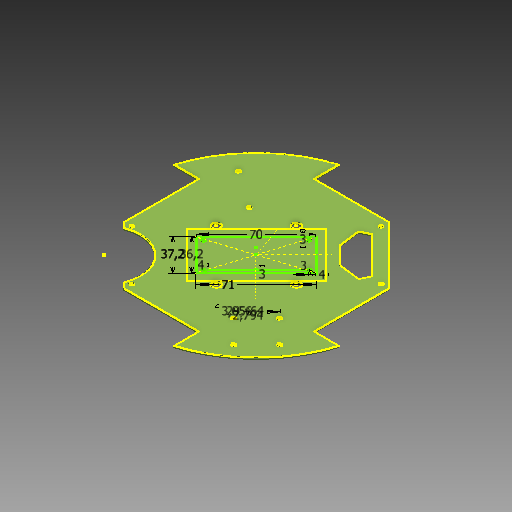
# Autodesk Inventor part: Board1.2
Saved by Autodesk Inventor 2020 (Build 240168000, 168)
## iProperties
Created: 2024-09-20
Part Number: Board1.2
Material: Типовые
Document SubType Name: Modeling
Designer: Ivan
Density: 1 g/cm^3
Appearance: Оливково-зеленый
Author: Ivan
Autodesk Inventor part; units mm, degrees
ref_plane "YZ Plane" through (0, 0, 0) normal (1, 0, 0) x (0, 1, 0)
ref_plane "XZ Plane" through (0, 0, 0) normal (0, 1, 0) x (-1, 0, 0)
ref_plane "XY Plane" through (0, 0, 0) normal (0, 0, 1) x (1, 0, 0)
sketch "Эскиз1" plane through (0, 0, 0) normal (0, 1, 0) x (-1, 0, 0)
  line L0 (-42.002343, -27.440424) -> (-27.440424, -42.002343)
  line L1 (-27.440424, -42.002343) -> (-25.169576, -59.537657)
  line L2 (-25.169576, -59.537657) -> (-32.692388, -63.237612)
  line L3 (-32.692388, -63.237612) -> (-63.237612, -32.692388)
  line L4 (-63.237612, -32.692388) -> (-59.537657, -25.169576)
  line L5 (-59.537657, -25.169576) -> (-42.002343, -27.440424)
  circle A0 centre (-72.43, 16) radius 3.3 construction
  circle A1 centre (44.87, -82.901522) radius 3.3 construction
  circle A2 centre (42.22, 16) radius 3.3
  circle A3 centre (-44.87, 82.901522) radius 3.3 construction
  circle A4 centre (-42.22, 16) radius 3.3 construction
  circle A5 centre (-82.901522, 44.87) radius 3.3 construction
  circle A6 centre (-16, 42.22) radius 3.3 construction
  circle A7 centre (72.43, -16) radius 3.3 construction
  circle A8 centre (16, -72.43) radius 3.3 construction
  circle A9 centre (-16, -72.43) radius 3.3 construction
  circle A10 centre (-42.22, -16) radius 3.3 construction
  circle A11 centre (16, -42.22) radius 3.3 construction
  circle A12 centre (16, 42.22) radius 3.3
  circle A13 centre (16, 72.43) radius 3.3 construction
  circle A14 centre (42.22, -16) radius 3.3 construction
  circle A15 centre (72.43, 16) radius 3.3 construction
  circle A16 centre (-16, 72.43) radius 3.3 construction
  circle A17 centre (82.901522, -44.87) radius 3.3 construction
  circle A18 centre (-16, -42.22) radius 3.3 construction
  circle A19 centre (-72.43, -16) radius 3.3 construction
  line L6 (31, 78.772353) -> (-31, 78.772353)
  line L7 (-31, 78.772353) -> (-31, 99.272353)
  arc A20 (-31, 99.272353) -> (-99.272353, 31) centre (0, 0) ccw
  line L8 (-99.272353, 31) -> (-78.772353, 31)
  line L9 (-78.772353, 31) -> (-78.772353, -31)
  line L10 (-78.772353, -31) -> (-99.272353, -31)
  arc A21 (-99.272353, -31) -> (-98.086264, -34.57) centre (0, 0) ccw
  arc A22 (-34.57, -98.086264) -> (-98.086264, -34.57) centre (-109.02125, -109.02125) ccw
  arc A23 (-34.57, -98.086264) -> (-31, -99.272353) centre (0, 0) ccw
  line L11 (-31, -99.272353) -> (-31, -78.772353)
  line L12 (-31, -78.772353) -> (31, -78.772353)
  line L13 (31, -78.772353) -> (31, -99.272353)
  arc A24 (31, -99.272353) -> (99.272353, -31) centre (0, 0) ccw
  line L14 (99.272353, -31) -> (78.772353, -31)
  line L15 (78.772353, -31) -> (78.772353, 31)
  line L16 (78.772353, 31) -> (99.272353, 31)
  arc A25 (99.272353, 31) -> (98.086264, 34.57) centre (0, 0) ccw
  arc A26 (34.57, 98.086264) -> (98.086264, 34.57) centre (109.02125, 109.02125) ccw
  arc A27 (34.57, 98.086264) -> (31, 99.272353) centre (0, 0) ccw
  line L17 (31, 99.272353) -> (31, 78.772353)
  circle A28 centre (31, 72.43) radius 1.5
  circle A29 centre (72.43, 31) radius 1.5
  circle A30 centre (0, 0) radius 20
  circle A31 centre (-72.43, -31) radius 1.5
  circle A32 centre (-31, -72.43) radius 1.5
  line L18 (-55.861436, 32.526912) -> (-79.195959, 55.861436)
  line L19 (-79.195959, 55.861436) -> (-55.861436, 79.195959)
  line L20 (-55.861436, 79.195959) -> (-32.526912, 55.861436)
  line L21 (-32.526912, 55.861436) -> (-55.861436, 32.526912)
  line L22 (48.313848, -22.45283) -> (80.459207, -54.598189)
  line L23 (80.459207, -54.598189) -> (54.598189, -80.459207)
  line L24 (54.598189, -80.459207) -> (22.45283, -48.313848)
  line L25 (22.45283, -48.313848) -> (48.313848, -22.45283)
  line L26 (31, 78.772353) -> (78.772353, 31)
  circle A33 centre (31, 72.43) radius 3.5 construction
  circle A34 centre (72.43, 31) radius 1.5 construction
  circle A35 centre (72.43, 31) radius 3.5 construction
  arc A36 (35.373192, 74.399161) -> (74.399161, 35.373192) centre (63.193264, 63.193264) ccw
  line L27 (-47.729708, -10.253048) -> (10.253048, 47.729708)
  line L28 (10.253048, 47.729708) -> (47.729708, 10.253048)
  line L29 (47.729708, 10.253048) -> (-10.253048, -47.729708)
  line L30 (-10.253048, -47.729708) -> (-47.729708, -10.253048)
  line L31 (-32.526912, 55.861436) -> (-55.861436, 32.526912) construction
  line L32 (-47.729708, -10.253048) -> (47.729708, 10.253048) construction
  line L33 (-78.772353, -31) -> (-31, -78.772353)
  dimension "d0" = 7
  dimension "d1" = 7
  dimension "d2" = 82
  dimension "d3" = 53
  constraints: 68 end point, 37 centre point, 18 point on circle, 4 coincident, 3 parallel, 2 point on line, 2 tangent, 1 midpoint, 1 perpendicular
  measures "d0" diameter of A33
  measures "d1" diameter of A35
  measures "d2" distance of L28.end L29.end
  measures "d3" distance of L27.end L28.end
extrude "Выдавливание1" add sketch "Эскиз1" along normal blind 1.6 contours A2 L28 | L28 A12 | L26 A36 L15 L14 A24 L13 L12 L33 L9 L8 A20 L7 L6 | L18 L19 L20 L21 | L22 L23 L24 L25 picked at (43.146155, 15.474263) picked at (17.150343, 42.083412)
sketch "Эскиз2" plane through (0, 0, 0) normal (0, 1, 0) x (1, 0, 0)
  circle A0 centre (26.769578, -48.318655) radius 1.397
  circle A1 centre (47.603772, -27.484461) radius 1.397
  line L0 (47.603772, -27.484461) -> (26.769578, -48.318655) construction
  line L1 (22.45283, -48.313848) -> (24.613608, -50.474625) construction
  line L2 (26.769578, -48.318655) -> (24.613608, -50.474625) construction
  line L3 (-47.729708, -10.253048) -> (10.253048, 47.729708)
  line L4 (47.729708, 10.253048) -> (-10.253048, -47.729708)
  point P0 (-22.45283, 48.313848)
  point P1 (-79.195959, 55.861436)
  point P2 (79.195959, -55.861436)
  dimension "d6" = 3.0558
  dimension "d8" = 29.464
  dimension "d9" = 2.794
  constraints: 6 end point, 2 centre point, 1 collinear, 1 equal radius, 1 perpendicular
  measures "d6" distance from line of L0 L1.start
  measures "d8" distance of L0.start L0.end
  measures "d9" diameter of A0
sketch "Эскиз4" plane through (0, 1.6, 0) normal (0, 1, 0) x (1, 0, 0)
  arc A0 (75.513396, -56.886374) -> (75.513396, -52.643733) centre (73.392076, -54.765053) ccw
  line L0 (75.513396, -52.643733) -> (57.12862, -34.258957)
  arc A1 (57.12862, -34.258957) -> (52.885979, -34.258957) centre (55.007299, -36.380277) ccw
  line L1 (52.885979, -34.258957) -> (34.501203, -52.643733)
  arc A2 (34.501203, -52.643733) -> (34.501203, -56.886374) centre (36.622523, -54.765053) ccw
  line L2 (34.501203, -56.886374) -> (52.885979, -75.27115)
  arc A3 (52.885979, -75.27115) -> (57.12862, -75.27115) centre (55.007299, -73.14983) ccw
  line L3 (57.12862, -75.27115) -> (75.513396, -56.886374)
  circle A4 centre (62.785474, -48.754646) radius 0.5
  circle A5 centre (55.007299, -73.856937) radius 1.6
  circle A6 centre (74.099182, -54.765053) radius 1.6
  circle A7 centre (55.007299, -35.67317) radius 1.6
  circle A8 centre (61.017707, -39.915811) radius 0.5
  circle A9 centre (55.714406, -41.683578) radius 0.5
  circle A10 centre (57.482173, -43.451345) radius 0.5
  circle A11 centre (59.24994, -45.219112) radius 0.5
  circle A12 centre (61.017707, -46.986879) radius 0.5
  circle A13 centre (43.693591, -64.310995) radius 0.5
  circle A14 centre (41.925824, -62.543228) radius 0.5
  circle A15 centre (62.785474, -41.683578) radius 0.5
  circle A16 centre (59.24994, -38.148044) radius 0.5
  circle A17 centre (53.946639, -39.915811) radius 0.5
  circle A18 centre (35.915416, -54.765053) radius 1.6
  circle A19 centre (40.158057, -60.775461) radius 0.5
  circle A20 centre (38.39029, -59.007694) radius 0.5
  circle A21 centre (64.553241, -50.522413) radius 0.5
  circle A22 centre (66.321008, -45.219112) radius 0.5
  circle A23 centre (64.553241, -43.451345) radius 0.5
  circle A24 centre (68.088775, -46.986879) radius 0.5
  circle A25 centre (69.856542, -48.754646) radius 0.5
  circle A26 centre (71.624309, -50.522413) radius 0.5
  line L4 (47.729708, 10.253048) -> (-10.253048, -47.729708)
  line L5 (18.73833, -18.73833) -> (73.539105, -73.539105) construction
  arc A27 (31, -99.272353) -> (99.272353, -31) centre (0, 0) ccw
  line L6 (-31, -78.772353) -> (31, -78.772353)
  line L7 (78.772353, -31) -> (31, -78.772353) construction
  point P0 (55.007299, -54.765053)
  point P1 (54.886176, -54.886176)
  constraints: 27 centre point, 12 end point, 9 point on circle, 2 midpoint, 1 point on line
extrude "Выдавливание4" cut sketch "Эскиз4" against normal through all contours A5 | A6 | A7 | A18
sketch "Эскиз5" plane through (0, 0, 0) normal (0, -1, 0) x (1, 0, 0)
  circle A0 centre (-37.246198, -31.292358) radius 1.6
  circle A1 centre (-67.882251, -53.033009) radius 1.6
  arc A2 (99.272353, 31) -> (31, 99.272353) centre (0, 0) ccw
  constraints: 3 centre point, 2 point on circle
extrude "Выдавливание5" cut sketch "Эскиз5" against normal through all
sketch "Эскиз6" plane through (0, 1.6, 0) normal (0, 1, 0) x (1, 0, 0)
  circle A0 centre (49.151483, 117.512898) radius 1.65
  circle A1 centre (49.151483, 117.512898) radius 3.35
  circle A2 centre (3.90139, 156.848367) radius 1.65
  circle A3 centre (79.999989, 152.999936) radius 1.65
  circle A4 centre (34.74993, 192.33537) radius 1.65
  circle A5 centre (41.950689, 154.924131) radius 41.494038
  line L0 (45.976694, 118.582111) -> (51.702547, 119.684205)
  arc A6 (39.303109, 113.514645) -> (45.976694, 118.582111) centre (26.737362, 136.991182) ccw
  arc A7 (51.702547, 119.684205) -> (59.780333, 117.456035) centre (62.733836, 143.919668) ccw
  arc A8 (78.499345, 155.995027) -> (82.588741, 163.308869) centre (57.591924, 172.485191) ccw
  circle A9 centre (79.999989, 152.999936) radius 3.35
  arc A10 (81.535526, 142.482434) -> (78.204844, 150.171517) centre (55.740492, 135.874711) ccw
  arc A11 (5.402031, 153.853275) -> (1.312636, 146.539393) centre (26.309482, 137.363149) ccw
  circle A12 centre (3.90139, 156.848367) radius 3.35
  arc A13 (2.365865, 167.365871) -> (5.696538, 159.676785) centre (28.160906, 173.973566) ccw
  arc A14 (32.198864, 190.164066) -> (24.121078, 192.392253) centre (21.16753, 165.928649) ccw
  circle A15 centre (34.74993, 192.33537) radius 3.35
  arc A16 (44.598268, 196.333616) -> (37.924718, 191.266155) centre (57.164078, 172.857113) ccw
  line L1 (39.303109, 113.514645) -> (59.780333, 117.456035) construction
  line L2 (-47.022601, -10.253048) -> (10.253048, 47.022601) construction
  line L3 (2.365865, 167.365871) -> (59.780333, 117.456035) construction
  line L4 (24.121036, 192.392233) -> (81.535512, 142.48239) construction
  line L5 (1.312636, 146.539393) -> (44.598268, 196.333616) construction
  line L6 (82.588741, 163.308869) -> (39.303109, 113.514645) construction
  circle A17 centre (41.950689, 154.924131) radius 38.097924 construction
  line L7 (45.976694, 118.582111) -> (46.911064, 113.727652) construction
  line L8 (78.204844, 150.171517) -> (78.499345, 155.995027) construction
  line L9 (41.950689, 154.924131) -> (79.999989, 152.999936) construction
  line L10 (41.950689, 154.924131) -> (34.74993, 192.33537) construction
  line L11 (41.950689, 154.924131) -> (3.90139, 156.848367) construction
  line L12 (5.696538, 159.676785) -> (5.402031, 153.853275) construction
  line L13 (32.198864, 190.164066) -> (37.924718, 191.266155) construction
  line L14 (41.950689, 154.924131) -> (49.151483, 117.512898) construction
  circle A18 centre (-37.822435, 4.573567) radius 3.3
  circle A19 centre (-4.573567, 37.822435) radius 3.3
  circle A20 centre (4.573567, -37.822435) radius 3.3
  circle A21 centre (37.822435, -4.573567) radius 3.3
  circle A22 centre (16, -49.72) radius 3.3
  line L15 (-37.822435, 4.573567) -> (-4.573567, 37.822435) construction
  line L16 (4.573567, -37.822435) -> (37.822435, -4.573567) construction
  line L17 (-21.198001, 21.198001) -> (21.198001, -21.198001) construction
  line L18 (-4.573567, 37.822435) -> (37.822435, -4.573567) construction
  point P0 (-47.616756, 71.930474)
  point P1 (-60.382397, 55.652797)
  point P2 (-60.382397, 22.39343)
  point P3 (-47.616756, 6.115753)
  point P4 (2.783098, 6.115753)
  point P5 (15.548739, 22.39343)
  point P6 (15.244077, 55.858669)
  point P7 (2.910415, 71.585522)
  point P8 (0, 0)
  point P9 (-47.616756, 71.930474)
  point P10 (-60.382397, 55.652797)
  point P11 (-60.382397, 22.39343)
  point P12 (-47.616756, 6.115753)
  point P13 (2.783098, 6.115753)
  point P14 (15.548739, 22.39343)
  point P15 (15.244077, 55.858669)
  point P16 (2.910415, 71.585522)
  point P17 (0, 0)
  dimension "d45" = 82.98808
  dimension "d43" = 3.3
  dimension "d44" = 6.7
  dimension "d46" = 26.62791
  dimension "d47" = 20.47722
  dimension "d48" = 3.71477
  dimension "d49" = 33.16031
  dimension "d50" = 50.33796
  dimension "d51" = 16.58016
  dimension "d52" = 25.16898
  dimension "d53" = 10.42652
  dimension "d54" = 10.42652
  dimension "d55" = 10.42652
  dimension "d56" = 10.42652
  dimension "d57" = 10.42652
  dimension "d58" = 10.42652
  dimension "d59" = 59.957
  dimension "d60" = 47.021
  constraints: 38 end point, 28 point on circle, 22 centre point, 13 equal radius, 9 perpendicular, 6 coincident, 4 equal length, 4 parallel, 3 midpoint, 1 tangent, 12 other
  measures "d43" diameter of A0
  measures "d44" diameter of A1
  measures "d46" radius of A6
  measures "d47" horizontal distance of L1.end L1.start
  measures "d48" distance from line of L1 L0.start
  measures "d49" distance from line of L4 L3.start
  measures "d50" distance from line of L5 L6.start
  measures "d51" distance from line of L3 point (41.951, 154.924)
  measures "d52" distance from line of L5 point (41.951, 154.924)
  measures "d53" distance from line of L9 L6.start
  measures "d54" distance from line of L9 A10.start
  measures "d55" distance from line of L10 A14.end
  measures "d56" distance from line of L10 L5.end
  measures "d57" distance from line of L11 L3.start
  measures "d58" distance from line of L14 L1.end
  measures "d59" distance from line of L15 L16.end
  measures "d60" distance from line of L18 L15.start
extrude "Выдавливание6" cut sketch "Эскиз6" against normal blind 10 contours A18 | A19 | A20 | A21
sketch "Эскиз7" plane through (0, 1.6, 0) normal (0, 1, 0) x (1, 0, 0)
  line L0 (-38.254477, -11.950105) -> (-11.950105, -38.254477)
  line L1 (-11.950105, -38.254477) -> (38.254477, 11.950105)
  line L2 (38.254477, 11.950105) -> (11.950105, 38.254477)
  line L3 (11.950105, 38.254477) -> (-38.254477, -11.950105)
  line L4 (-38.254477, -11.950105) -> (38.254477, 11.950105) construction
  line L5 (-11.950105, -38.254477) -> (11.950105, 38.254477) construction
  line L6 (47.022601, 10.253048) -> (-10.253048, -47.022601) construction
  line L7 (-47.729708, -10.253048) -> (10.253048, 47.729708)
  line L8 (-10.253048, -47.729708) -> (-47.729708, -10.253048)
  line L9 (10.253048, 47.729708) -> (47.729708, 10.253048)
  line L10 (47.729708, 10.253048) -> (-10.253048, -47.729708)
  line L11 (-38.254477, -11.950105) -> (-11.950105, -38.254477)
  line L12 (-11.950105, -38.254477) -> (38.254477, 11.950105)
  line L13 (38.254477, 11.950105) -> (11.950105, 38.254477)
  line L14 (11.950105, 38.254477) -> (-38.254477, -11.950105)
  line L15 (-38.254477, -11.950105) -> (38.254477, 11.950105) construction
  line L16 (-11.950105, -38.254477) -> (11.950105, 38.254477) construction
  line L17 (47.022601, 10.253048) -> (-10.253048, -47.022601) construction
  line L18 (37.54737, 11.950105) -> (11.950105, 37.54737)
  line L19 (11.950105, 37.54737) -> (-37.54737, -11.950105)
  line L20 (-37.54737, -11.950105) -> (-11.950105, -37.54737)
  line L21 (-11.950105, -37.54737) -> (37.54737, 11.950105)
  line L22 (37.54737, 11.950105) -> (-37.54737, -11.950105) construction
  line L23 (32.597623, 11.242998) -> (-11.242998, -32.597623)
  line L24 (0, 0) -> (31.732181, -31.732181) construction
  circle A0 centre (32.597623, 11.242998) radius 1.5
  line L25 (0, 0) -> (31.732181, 31.732181) construction
  line L26 (0, 0) -> (-9.9, 29) construction
  circle A1 centre (11.242998, 32.597623) radius 1.5
  circle A2 centre (-11.242998, -32.597623) radius 1.5
  circle A3 centre (-32.597623, -11.242998) radius 1.5
  point P0 (0, 0)
  point P1 (0, 0)
  point P2 (10.677312, -10.677312)
  point P3 (-4.979708, 4.979708)
  point P4 (0, 0)
  dimension "d63" = 37.2
  dimension "d64" = 71
  dimension "d67" = 37.2
  dimension "d68" = 71
  dimension "d69" = 36.2
  dimension "d70" = 70
  dimension "d71" = 4
  dimension "d72" = 3
  dimension "d73" = 3
  dimension "d74" = 3
  dimension "d75" = 4
  constraints: 46 end point, 10 parallel, 9 midpoint, 5 coincident, 4 centre point, 4 perpendicular, 3 symmetric about line, 2 point on line, 4 other
  measures "d63" distance of L0.start L0.end
  measures "d64" distance from line of L0 L1.end
  measures "d67" distance of L11.start L11.end
  measures "d68" distance from line of L11 L12.end
  measures "d69" distance of L20.end L19.end
  measures "d70" distance of L19.end L18.end
  measures "d71" distance from line of L18 L23.start
  measures "d72" distance from line of L21 point (10.677, -10.677)
  measures "d73" diameter of A0
  measures "d74" distance from line of L19 A1.centre
  measures "d75" distance from line of L20 L23.end
extrude "Выдавливание8" add sketch "Эскиз7" against normal up to surface (1.6 mm away) contours L3 L2 L1 L0 | L7 L9 L10 L8 | L21 L20 L19 L18 | A0 | A1 | A2 | A3
hole "Отверстие1" at (-32.597623, 1.6, 11.242998) at (11.242998, 1.6, -32.597623) at (32.597623, 1.6, -11.242998) at (-11.242998, 1.6, 32.597623) direction (0, -1, 0) diameter 3 end through all
sketch "Эскиз8" plane through (0, 1.6, 0) normal (0, 1, 0) x (1, 0, 0)
  circle A0 centre (32.597623, 11.242998) radius 1.5
  circle A1 centre (-32.597623, -11.242998) radius 1.5
  circle A2 centre (11.242998, 32.597623) radius 1.5
  circle A3 centre (-11.242998, -32.597623) radius 1.5
  circle A4 centre (37.822435, -4.573567) radius 3.3
  circle A5 centre (-4.573567, 37.822435) radius 3.3
  circle A6 centre (4.573567, -37.822435) radius 3.3
  circle A7 centre (-37.822435, 4.573567) radius 3.3
  circle A8 centre (-37.246198, 31.292358) radius 1.6
  circle A9 centre (-67.882251, 53.033009) radius 1.6
  circle A10 centre (55.007299, -73.856937) radius 1.6
  circle A11 centre (74.099182, -54.765053) radius 1.6
  circle A12 centre (35.915416, -54.765053) radius 1.6
  circle A13 centre (55.007299, -35.67317) radius 1.6
  arc A14 (-31, 99.272353) -> (-99.272353, 31) centre (0, 0) ccw
  line L0 (-99.272353, 31) -> (-78.772353, 31)
  line L1 (-78.772353, 31) -> (-78.772353, -31)
  line L2 (-78.772353, -31) -> (-74.399161, -35.373192)
  arc A15 (-35.373192, -74.399161) -> (-74.399161, -35.373192) centre (-63.193264, -63.193264) ccw
  line L3 (-35.373192, -74.399161) -> (-31, -78.772353)
  line L4 (-31, -78.772353) -> (31, -78.772353)
  line L5 (31, -78.772353) -> (31, -99.272353)
  arc A16 (31, -99.272353) -> (99.272353, -31) centre (0, 0) ccw
  line L6 (99.272353, -31) -> (78.772353, -31)
  line L7 (78.772353, -31) -> (78.772353, 31)
  line L8 (78.772353, 31) -> (31, 78.772353)
  line L9 (31, 78.772353) -> (-31, 78.772353)
  line L10 (-31, 78.772353) -> (-31, 99.272353)
  circle A17 centre (31, 72.43) radius 1.5
  circle A18 centre (-72.43, -31) radius 1.5
  line L11 (42.002343, 27.440424) -> (27.440424, 42.002343)
  line L12 (27.440424, 42.002343) -> (25.169576, 59.537657)
  line L13 (25.169576, 59.537657) -> (32.692388, 63.237612)
  line L14 (32.692388, 63.237612) -> (63.237612, 32.692388)
  line L15 (63.237612, 32.692388) -> (59.537657, 25.169576)
  line L16 (59.537657, 25.169576) -> (42.002343, 27.440424)
  circle A19 centre (-31, -72.43) radius 1.5
  circle A20 centre (72.43, 31) radius 1.5
equation "\"d53\" = d58"
equation "\"d54\" = d58"
equation "\"d55\" = d58"
equation "\"d56\" = d58"
equation "\"d57\" = d58"
